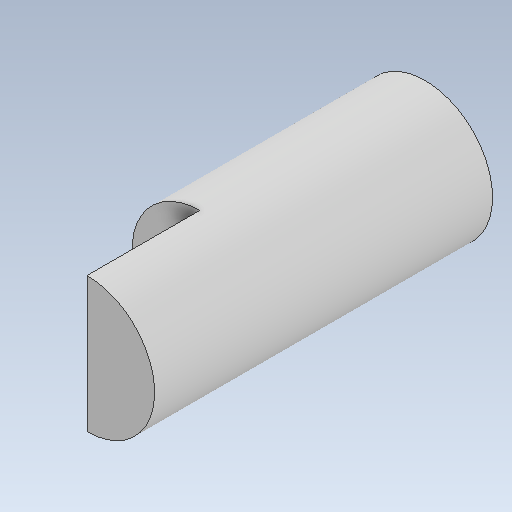
# Autodesk Inventor part: apoio tras sensor
Saved by Autodesk Inventor 2020 (Build 240168000, 168)
## iProperties
Created: 2020-05-13
Part Number: apoio tras sensor
Material: Genérico
Document SubType Name: Modeling
Designer: gi-se
Density: 1 g/cm^3
Appearance: Padrão
Author: gi-se
Autodesk Inventor part; units mm, degrees
ref_plane "YZ Plane" through (0, 0, 0) normal (1, 0, 0) x (0, 1, 0)
ref_plane "XZ Plane" through (0, 0, 0) normal (0, 1, 0) x (-1, 0, 0)
ref_plane "XY Plane" through (0, 0, 0) normal (0, 0, 1) x (1, 0, 0)
sketch "Esboço1" plane through (0, 0, 0) normal (0, 0, 1) x (1, 0, 0)
  circle A0 centre (0, 32) radius 2.4 projected
  line L0 (0, 29.6) -> (0, 34.4)
  point P0 (0, 0)
  constraints: 2 end point, 2 point on circle, 1 vertical
extrude "Extrusão1" add sketch "Esboço1" against normal blind 8
sketch "Esboço2" plane through (0, 32, 0) normal (0, 0, 1) x (1, 0, 0)
  circle A0 centre (0, 0) radius 2.4 projected
  line L0 (0, -2.4) -> (0, 2.4)
  point P0 (0, -32)
  constraints: 2 end point, 2 point on circle, 1 vertical
extrude "Extrusão2" add sketch "Esboço2" along normal blind 4 contours A0 L0 picked at (0.4988, 0.6255)
